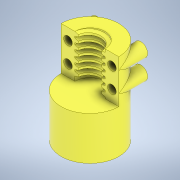
# Autodesk Inventor part: SpindleAdaptor_A_V4_Wide
Saved by Autodesk Inventor 2022.2 (Build 262287000, 287)
## iProperties
Created: 2022-11-20
Part Number: SpindleAdaptor_A_V4_Wide
Material: ABS Plastic
Document SubType Name: Modeling
Designer: jaege
Density: 1.06 g/cm^3
Appearance: Smooth - Yellow
Mass: 4.16051 g
Surface Area: 27.1261 cm^2
Volume: 4.16051 cm^3
Author: jaege
## iProperties of the stored document SpindleAdaptor_A_V2_3DPrint.ipt
Created: 2022-11-23
Part Number: SpindleAdaptor_A_V2_3DPrint
Material: Generic
Document SubType Name: Modeling
Designer: jaege
Density: 1 g/cm^3
Appearance: Default
Author: jaege
Autodesk Inventor part; units mm, degrees
ref_plane "YZ Plane" through (0, 0, 0) normal (1, 0, 0) x (0, 1, 0)
ref_plane "XZ Plane" through (0, 0, 0) normal (0, 1, 0) x (-1, 0, 0)
ref_plane "XY Plane" through (0, 0, 0) normal (0, 0, 1) x (1, 0, 0)
sketch "Sketch1" plane through (0, 0, 0) normal (0, 1, 0) x (-1, 0, 0)
  circle A0 centre (0, 0) radius 10
  dimension "d0" = 20
  constraints: 1 centre point, 1 coincident
  measures "d0" diameter of A0
extrude "Extrusion1" add sketch "Sketch1" along normal blind 30
sketch "Sketch2" plane through (0, 30, 0) normal (0, 1, 0) x (1, 0, 0)
  circle A0 centre (0, 0) radius 5.25
  dimension "d3" = 10.5
  constraints: 1 centre point, 1 coincident
  measures "d3" diameter of A0
extrude "Extrusion2" cut sketch "Sketch2" against normal blind 15
sketch "Sketch3" plane through (0, 0, 0) normal (0, 0, 1) x (1, 0, 0)
  line L0 (10, 30) -> (-10, 30) projected
  line L1 (10, 0) -> (-10, 0) projected
  line L2 (-5.25, 15) -> (5.25, 15) projected
  line L3 (-5.25, 30) -> (5.25, 30) projected
  line L4 (-5.25, 30) -> (-5.25, 15) projected
  line L5 (5.25, 30) -> (5.25, 15) construction
  line L6 (-5.25, 15) -> (5.25, 15) projected
  line L7 (-4, 15) -> (4, 15) construction
  line L8 (4, 15) -> (4, 30) construction
  line L9 (4, 30) -> (-4, 30) construction
  line L10 (-4, 30) -> (-4, 15) construction
  line L11 (5.25, 30) -> (4, 29.6651)
  line L12 (2.634, 29.299) -> (4, 28.933) construction
  line L13 (4, 29.6651) -> (4, 28.933)
  line L14 (5.25, 28.5981) -> (5.25, 28)
  line L15 (5.25, 28) -> (4, 27.6651)
  line L16 (2.634, 27.299) -> (4, 26.933) construction
  line L17 (4, 29.6651) -> (2.634, 29.299) construction
  line L18 (4, 27.6651) -> (2.634, 27.299) construction
  line L19 (4, 28.933) -> (5.25, 28.5981)
  line L20 (4, 26.933) -> (5.25, 26.5981)
  line L21 (4, 27.6651) -> (4, 26.933)
  line L22 (5.25, 30) -> (5.25, 28.5981)
  line L23 (0, 30) -> (0, 15)
  point P0 (0, 0)
  point P1 (4, 29.299)
  dimension "d6" = 8
  dimension "d7" = 30
  dimension "d8" = 30
  dimension "d9" = 1.25
  dimension "d10" = 105
  dimension "d11" = 105
  dimension "d12" = 0.732
  dimension "d13" = 0.5981
  constraints: 34 end point, 9 point on line, 6 collinear, 3 midpoint, 2 parallel, 2 vertical, 1 horizontal, 1 perpendicular, 1 vertical alignment
  measures "d6" distance between parallel lines of L8 L10
  measures "d7" angle of L12 L11
  measures "d8" angle of L16 L15
  measures "d9" distance between parallel lines of L5 L13
  measures "d10" angle of L5 L11
  measures "d11" angle of L14 L15
  measures "d12" distance of L13.start L12.end
  measures "d13" distance of L14.start L14.end
coil "Coil1" sketch "Sketch3" operation add axis through (0, 30, 0) along (0, -1, 0) pitch 2 turns 7 hand right contours L22 L19 L13 L11
sketch "Sketch4" plane through (0, 0, 0) normal (0, -1, 0) x (1, 0, 0)
  circle A0 centre (0, 0) radius 3
  line L0 (-3, -3) -> (3, -3)
  line L1 (3, -3) -> (3, 2.5)
  line L2 (3, 2.5) -> (-3, 2.5)
  line L3 (-3, 2.5) -> (-3, -3)
  point P0 (1.6583, 2.5)
  point P1 (-1.6583, 2.5)
  dimension "d22" = 6
  dimension "d23" = 5.5
  constraints: 8 end point, 3 tangent, 2 parallel, 1 centre point, 1 coincident, 1 horizontal, 1 perpendicular
  measures "d22" diameter of A0
  measures "d23" distance of L0.end L1.end
extrude "Extrusion3" cut sketch "Sketch4" against normal blind 10 contours A0 L2 picked at (0.5528, -1.1165)
sketch "Sketch5" plane through (0, 0, 0) normal (0, 0, 1) x (1, 0, 0)
  line L0 (10, 30) -> (-10, 30) projected
  line L1 (-5.25, 15) -> (5.25, 15) projected
  line L2 (0, -6) -> (0, 36) projected
  line L3 (-7.625, 26) -> (-10, 26) construction
  line L4 (-7.625, 26) -> (-5.25, 26) construction
  line L5 (-5.25, 30) -> (-5.25, 15) projected
  line L6 (-10, 0) -> (-10, 30) projected
  circle A0 centre (-7.625, 19) radius 1.5
  circle A1 centre (-7.625, 26) radius 1.5
  circle A2 centre (7.625, 26) radius 1.5
  circle A3 centre (7.625, 19) radius 1.5
  point P0 (0, 0)
  point P1 (1.5921, 15)
  dimension "d26" = 4
  dimension "d27" = 4
  dimension "d28" = 3
  constraints: 4 centre point, 4 coincident, 4 end point, 4 vertical alignment, 3 equal radius, 2 horizontal, 2 horizontal alignment, 1 collinear, 1 symmetric about line
  measures "d26" distance from line of L0 L3.start
  measures "d27" distance from line of L1 point (-7.625, 19)
  measures "d28" diameter of A0
extrude "Extrusion4" cut sketch "Sketch5" along normal through all both and the other way through all contours A0 | A1 | A2 | A3
ref_plane "Work Plane1" through (0, 0, -10) normal (0, 0, -1) x (-1, 0, 0)
sketch "Sketch6" plane through (0, 0, -10) normal (0, 0, -1) x (-1, 0, 0)
  circle A0 centre (-7.625, 26) radius 1.5
  line L0 (-10, 0) -> (-10, 30) projected
  line L1 (-5.25, 28.5981) -> (-5.25, 30) projected
  line L2 (10, 0) -> (10, 30) projected
  line L3 (10, 30) -> (-10, 30) projected
  line L4 (0, 30) -> (0, 0)
  line L5 (-7.625, 26) -> (-7.625, 29.0718) construction
  line L6 (-7.625, 29.0718) -> (-10, 29.0718) construction
  line L7 (-7.625, 29.0718) -> (-5.25, 29.0718) construction
  line L8 (-5.25, 15) -> (5.25, 15) projected
  circle A1 centre (-7.625, 19) radius 1.5
  circle A2 centre (7.625, 19) radius 1.5
  circle A3 centre (7.625, 26) radius 1.5
  circle A4 centre (7.625, 19) radius 2.375
  circle A5 centre (7.625, 26) radius 2.375
  circle A6 centre (-7.625, 26) radius 2.375
  circle A7 centre (-7.625, 19) radius 2.375
  line L9 (-5.25, 28.5981) -> (-5.25, 0) construction
  line L10 (10, 0) -> (-10, 0) projected
  point P0 (-1.5921, 15)
  dimension "d31" = 3
  dimension "d32" = 4
  dimension "d33" = 4
  dimension "d34" = 4.75
  constraints: 10 end point, 8 centre point, 6 equal radius, 4 point on line, 3 coincident, 3 vertical, 2 horizontal alignment, 2 vertical alignment, 1 collinear, 1 midpoint, 1 perpendicular, 1 symmetric about line
  measures "d31" diameter of A0
  measures "d32" distance from line of L5.start L3
  measures "d33" distance from line of L8 A1.centre
  measures "d34" diameter of A7
ref_plane "Work Plane2" through (0, 0, 10) normal (0, 0, -1) x (-1, 0, 0)
extrude "Extrusion5" add sketch "Sketch6" against normal up to surface (20 mm away) contours A6 | A7 | A4 | A5
sketch "Sketch7" plane through (0, 30, 0) normal (0, 1, 0) x (1, 0, 0)
  line L0 (-5.25, 10) -> (-10, 10) projected
  circle A0 centre (0, 0) radius 5.25 projected
  circle A1 centre (0, 0) radius 10 projected
  line L1 (10, 10) -> (5.25, 10) projected
  line L2 (-10, 10) -> (-10, 0) projected
  line L3 (-5.25, 10) -> (-5.25, 8.511) projected
  line L4 (-10, -10) -> (-5.25, -10) projected
  line L5 (5.25, -10) -> (10, -10) projected
  line L6 (10, 0) -> (10, -10) projected
  line L7 (5.25, -8.511) -> (5.25, -10) projected
  line L8 (-5.25, -8.511) -> (-5.25, -10) projected
  line L9 (-10, 0) -> (-10, -10) projected
  circle A2 centre (0, 0) radius 10 projected
  line L10 (-10, 0) -> (10, 0)
  line L11 (-10, 0) -> (-10, 10)
  line L12 (-10, 10) -> (10, 10)
  line L13 (10, 10) -> (10, 0)
  point P0 (5.25, 0)
  point P1 (-5.25, -8.511)
  point P2 (10, 10)
  point P3 (5.25, 10)
  point P4 (-5.25, 10)
  constraints: 8 end point, 3 perpendicular, 1 collinear, 1 horizontal alignment, 1 tangent, 1 vertical, 5 other
extrude "Extrusion6" cut sketch "Sketch7" against normal up to surface (15 mm away) contours L3 A1 L2 L0 | L12 A1 L3 | A1 L10 A0 | L12 L1 L13 A1 | A0 L10 picked at (8.3331, 0.7417) picked at (1.5495, 0.8133)
thicken "Thicken1" operation add thickness 0.05 both sides no extend neighbours yes toward (0.988644, 0, -0.1502765) faces at (2.9659, 3.3333, -0.4508) (0.5528, 6.6667, 2.5)
body "Solid1"
